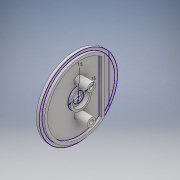
# Autodesk Inventor part: turn2Part
Saved by Autodesk Inventor 2018 (Build 220112000, 112)
## iProperties
Created: 2019-10-09
Part Number: turn2Part
Material: 一般
Document SubType Name: Modeling
Designer: Eiji Nishizawa
Density: 1 g/cm^3
Appearance: 既定
Mass: 6.96165 g
Surface Area: 73.2581 cm^2
Volume: 6.96165 cm^3
Author: Eiji Nishizawa
Autodesk Inventor part; units mm, degrees
ref_plane "YZ Plane" through (0, 0, 0) normal (1, 0, 0) x (0, 1, 0)
ref_plane "XZ Plane" through (0, 0, 0) normal (0, 1, 0) x (-1, 0, 0)
ref_plane "XY Plane" through (0, 0, 0) normal (0, 0, 1) x (1, 0, 0)
sketch "スケッチ1" plane through (0, 0, 0) normal (1, 0, 0) x (0, 1, 0)
  circle A0 centre (0, 0) radius 28
  line L0 (16.8575, 19.7946) -> (16.8575, -19.7946)
  line L1 (14.8575, 18.8482) -> (14.8575, -18.8482)
  arc A1 (18.1557, 18.611) -> (18.8392, -17.9188) centre (0, 0) ccw
  arc A2 (14.8575, 18.8482) -> (14.8575, -18.8482) centre (0, 0) ccw
  arc A3 (16.8575, 19.7946) -> (18.1557, 18.611) centre (0, 0) ccw
  arc A4 (18.8392, -17.9188) -> (16.8575, -19.7946) centre (0, 0) ccw
  line L2 (16.8575, 19.7946) -> (16.8575, -19.7946)
  line L3 (21.8575, 17.5) -> (21.8575, -17.5)
  dimension "d0" = 56
  dimension "d1" = 2
  dimension "d2" = 2
  dimension "d3" = 2
  dimension "d4" = 35
  dimension "d5" = 5
  constraints: 12 point on circle, 8 end point, 5 centre point, 5 coincident, 3 vertical, 1 collinear
  measures "d0" diameter of A0
  measures "d1" radial gap between concentric circles of A0 A1
  measures "d2" radial gap between concentric circles of A1 A2
  measures "d3" distance between parallel lines of L1 L0
  measures "d4" distance of L3.start L3.end
  measures "d5" distance between parallel lines of L0 L3
extrude "押し出し1" add sketch "スケッチ1" against normal blind 2 contours A0 L3 A3 | L3 A3 A1 A0 | L3 A3 A1 L0 | A3 L3 | L0 A1 | L1 A2
extrude "押し出し2" add sketch "スケッチ1" along normal blind 2 contours L0 A1
sketch "スケッチ2" plane through (0, 0, 0) normal (1, 0, 0) x (0, 0, -1)
  circle A0 centre (0, 0) radius 3.75
  circle A1 centre (0, 0) radius 7.5
  dimension "d10" = 7.5
  dimension "d11" = 15
  constraints: 2 centre point, 2 coincident
  measures "d10" diameter of A0
  measures "d11" diameter of A1
extrude "押し出し3" cut sketch "スケッチ2" against normal blind 2 contours A0
extrude "押し出し4" add sketch "スケッチ2" along normal blind 2
sketch "スケッチ3" plane through (2, 0, 0) normal (1, 0, 0) x (0, 0, -1)
  circle A0 centre (0, 0) radius 6
  dimension "d16" = 12
  constraints: 1 centre point, 1 coincident
  measures "d16" diameter of A0
extrude "押し出し5" cut sketch "スケッチ3" against normal blind 2.9
sketch "スケッチ4" plane through (0, 0, 0) normal (1, 0, 0) x (0, 0, -1)
  circle A0 centre (-10.8, 0) radius 3
  circle A1 centre (10.8, 0) radius 3
  circle A2 centre (-10.8, 0) radius 1.5
  circle A3 centre (10.8, 0) radius 1.5
  circle A4 centre (0, 0) radius 3.75 projected
  dimension "d19" = 6
  dimension "d20" = 6
  dimension "d21" = 3
  dimension "d22" = 3
  dimension "d23" = 10.8
  dimension "d25" = 21.6
  dimension "d26" = 10.8
  constraints: 4 centre point, 2 coincident
  measures "d19" diameter of A0
  measures "d20" diameter of A1
  measures "d21" diameter of A2
  measures "d22" diameter of A3
  measures "d23" distance of A4.centre A0.centre
  measures "d25" distance of A1.centre A0.centre
  measures "d26" distance of A4.centre A1.centre
extrude "押し出し6" add sketch "スケッチ4" along normal blind 9.5 contours A0 | A1
